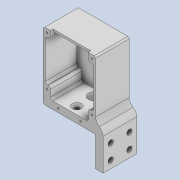
# Autodesk Inventor part: 0008-10-051 Cutie Priza
Saved by Autodesk Inventor 2020 (Build 240168000, 168)
## iProperties
Created: 2021-03-10
Part Number: 0008-10-051 Cutie Priza
Material: Generic
Document SubType Name: Modeling
Designer: Iulian Bors
Density: 1 g/cm^3
Appearance: Default
Description: Cutie priza
Mass: 164.87 g
Surface Area: 428.639 cm^2
Volume: 164.87 cm^3
Author: Iulian Bors
Subject: 051
Autodesk Inventor part; units mm, degrees
ref_plane "YZ Plane" through (0, 0, 0) normal (1, 0, 0) x (0, 1, 0)
ref_plane "XZ Plane" through (0, 0, 0) normal (0, 1, 0) x (-1, 0, 0)
ref_plane "XY Plane" through (0, 0, 0) normal (0, 0, 1) x (1, 0, 0)
sketch "Sketch1" plane through (0, 0, 0) normal (0, 0, 1) x (1, 0, 0)
  line L0 (-35, 45) -> (35, 45)
  line L1 (35, 45) -> (35, -45)
  line L2 (35, -45) -> (-35, -45)
  line L3 (-35, -45) -> (-35, 45)
  point P0 (0, 0)
  point P1 (0, 45)
  point P2 (-35, 0)
  dimension "d0" = 70
  dimension "d1" = 90
  constraints: 8 end point, 2 midpoint, 2 parallel, 1 horizontal, 1 horizontal alignment, 1 perpendicular, 1 vertical alignment
  measures "d0" distance of L0.start L0.end
  measures "d1" distance of L0.end L1.end
extrude "Extrusion1" add sketch "Sketch1" along normal blind 45
sketch "Sketch2" plane through (0, 0, 45) normal (0, 0, 1) x (1, 0, 0)
  line L0 (-25.3, 42) -> (25.3, 42)
  line L1 (25.3, 42) -> (25.3, -35)
  line L2 (25.3, -35) -> (-25.3, -35)
  line L3 (-25.3, -35) -> (-25.3, 42)
  line L4 (-35, 45) -> (-35, -45) projected
  line L5 (35, -45) -> (35, 45) projected
  line L6 (-35, -45) -> (35, -45) projected
  line L7 (35, 45) -> (-35, 45) projected
  point P0 (0, 0)
  dimension "d4" = 9.7
  dimension "d5" = 9.7
  dimension "d6" = 10
  dimension "d7" = 3
  constraints: 8 end point, 2 parallel, 1 horizontal, 1 perpendicular
  measures "d4" distance between parallel lines of L4 L3
  measures "d5" distance between parallel lines of L5 L1
  measures "d6" distance between parallel lines of L6 L2
  measures "d7" distance between parallel lines of L0 L7
extrude "Extrusion2" cut sketch "Sketch2" against normal blind 42 contours L0 L1 L2 L3
sketch "Sketch3" plane through (-35, 45, 0) normal (0, 1, 0) x (1, 0, 0)
  line L0 (60.3, -45) -> (9.7, -45)
  line L1 (9.7, -45) -> (9.7, -41.5)
  line L2 (9.7, -41.5) -> (60.3, -41.5)
  line L3 (60.3, -41.5) -> (60.3, -45)
  line L4 (9.7, -45) -> (9.7, -3) projected
  line L5 (60.3, -45) -> (60.3, -3) projected
  line L6 (70, -45) -> (0, -45) projected
  point P0 (35, 0)
  dimension "d10" = 3.5
  constraints: 8 end point, 3 collinear, 2 parallel, 1 horizontal, 1 perpendicular
  measures "d10" distance of L0.end L1.end
extrude "Extrusion3" cut sketch "Sketch3" against normal up to surface (3 mm away)
sketch "Sketch5" plane through (0, 0, 45) normal (0, 0, 1) x (1, 0, 0)
  line L0 (-33, 45) -> (-25, 45)
  line L1 (-25, 45) -> (25, 45)
  line L2 (25, 45) -> (33, 45)
  line L3 (33, 45) -> (35, 43)
  line L4 (35, 43) -> (35, -43)
  line L5 (35, -43) -> (33, -45)
  line L6 (33, -45) -> (-33, -45)
  line L7 (-33, -45) -> (-35, -43)
  line L8 (-35, -43) -> (-35, 43)
  line L9 (-35, 43) -> (-33, 45)
  line L10 (-25, -30) -> (-25, 45)
  line L11 (25, -30) -> (-25, -30)
  line L12 (25, 45) -> (25, -30)
  circle A0 centre (-30, 40) radius 2
  circle A1 centre (30, -25) radius 2
  circle A2 centre (-15, -40) radius 2
  circle A3 centre (15, -40) radius 2
  circle A4 centre (30, 40) radius 2
  circle A5 centre (-30, -25) radius 2
  line L13 (14.15, -21.6) -> (14.15, 28.85)
  arc A6 (14.15, 28.85) -> (11.65, 31.35) centre (11.65, 28.85) ccw
  line L14 (11.65, 31.35) -> (-12.5, 31.35)
  arc A7 (-12.5, 31.35) -> (-15, 28.85) centre (-12.5, 28.85) ccw
  line L15 (-15, 28.85) -> (-15, -21.6)
  arc A8 (-15, -21.6) -> (-12.5, -24.1) centre (-12.5, -21.6) ccw
  line L16 (-12.5, -24.1) -> (11.65, -24.1)
  arc A9 (11.65, -24.1) -> (14.15, -21.6) centre (11.65, -21.6) ccw
  circle A10 centre (20.135, 3.655) radius 2
  circle A11 centre (-19.865, 3.655) radius 2
  point P0 (0, 0)
  constraints: 34 end point, 12 centre point, 8 point on circle, 7 horizontal, 6 vertical, 48 other
hole "Hole2" at (-30, 40, 45) at (30, 40, 45) at (30, -25, 45) at (15, -40, 45) at (-15, -40, 45) at (-30, -25, 45) direction (0, 0, -1) diameter 2.459 depth 30 tip angle 118 thread size "M3x0.5" class "6H" standard "ISO Metric profile"
sketch "Sketch6" plane through (-25.3, -35, 45) normal (0, 1, 0) x (1, 0, 0)
  line L0 (50.6, 0) -> (0, 0) projected
  line L1 (0, 0) -> (0, 42) projected
  line L2 (50.6, 0) -> (50.6, 42) projected
  point P0 (25.3, 45)
  point P1 (10, 10)
  point P2 (25.3, 10)
  point P3 (25.3, 0)
  dimension "d30" = 10
  dimension "d31" = 10
  constraints: 1 horizontal alignment, 1 midpoint, 1 vertical alignment
  measures "d30" distance from line of L0 point (10, 10)
  measures "d31" distance from line of L1 point (10, 10)
hole "Hole3" at (0, -35, 35) direction (0, -1, 0) diameter 6 end through all countersink diameter 12 countersink angle 90
sketch "Sketch8" plane through (35, -45, 0) normal (1, 0, 0) x (0, 0, -1)
  line L0 (-45, 10) -> (0, 10)
  line L1 (0, 10) -> (0, -40)
  line L2 (0, -40) -> (-45, -40)
  line L3 (-45, -40) -> (-45, 10)
  line L4 (0, 0) -> (-45, 0) projected
  line L5 (-45, 0) -> (-45, 90) projected
  line L6 (0, 0) -> (0, 90) projected
  circle A0 centre (-35, -10) radius 3.5
  circle A1 centre (-10, -10) radius 3.5
  circle A2 centre (-35, -30) radius 3.5
  circle A3 centre (-10, -30) radius 3.5
  point P0 (0, 45)
  dimension "d42" = 10
  dimension "d43" = 40
  dimension "d44" = 7
  dimension "d45" = 7
  dimension "d46" = 10
  dimension "d47" = 10
  dimension "d48" = 10
  dimension "d59" = 10
  constraints: 8 end point, 4 centre point, 2 collinear, 2 equal radius, 2 horizontal alignment, 2 parallel, 2 vertical alignment, 1 horizontal, 1 perpendicular
  measures "d42" distance between parallel lines of L4 L0
  measures "d43" distance between parallel lines of L4 L2
  measures "d44" diameter of A0
  measures "d45" diameter of A1
  measures "d46" distance from line of A0.centre L3
  measures "d47" distance from line of L1 A1.centre
  measures "d48" distance from line of L4 A0.centre
  measures "d59" distance from line of L2 A2.centre
extrude "Extrusion4" add sketch "Sketch8" along normal blind 10
fillet "Fillet1" radius 10 2 edges at (35, -35, 22.5) (45, -35, 22.5)
chamfer "Chamfer2" distance 2 angle 45 3 edges at (35, 45, 22.5) (-35, 45, 22.5) (-35, -45, 22.5)
sketch "Sketch9" plane through (-25.3, -35, 45) normal (0, 1, 0) x (1, 0, 0)
  circle A0 centre (25.3, 33) radius 7.5
  line L0 (50.6, 42) -> (0, 42) projected
  point P0 (25.3, 45)
  point P1 (25.3, 42)
  dimension "d55" = 15
  dimension "d56" = 9
  constraints: 1 centre point, 1 midpoint, 1 vertical alignment
  measures "d55" diameter of A0
  measures "d56" distance from line of A0.centre L0
extrude "Extrusion5" cut sketch "Sketch9" against normal through all
sketch "Sketch10" plane through (0, 0, 45) normal (0, 0, 1) x (1, 0, 0)
  line L0 (-32, 35) -> (32, 35)
  line L1 (32, 35) -> (32, -20)
  line L2 (32, -20) -> (-32, -20)
  line L3 (-32, -20) -> (-32, 35)
  line L4 (-25.3, -35) -> (-25.3, 45) projected
  line L5 (-35, 43) -> (-35, -43) projected
  circle A0 centre (-30, 40) radius 1.2295 projected
  circle A1 centre (-30, -25) radius 1.2295 projected
  point P0 (0, 0)
  point P1 (0, 35)
  point P2 (-32, 7.5)
  dimension "d60" = 3
  dimension "d61" = 5
  dimension "d62" = 5
  constraints: 8 end point, 2 midpoint, 2 parallel, 1 horizontal, 1 perpendicular, 1 vertical alignment
  measures "d60" distance between parallel lines of L5 L3
  measures "d61" distance from line of A0.centre L0
  measures "d62" distance from line of A1.centre L2
extrude "Extrusion6" cut sketch "Sketch10" against normal up to surface (42 mm away) contours L0 L4 L2 L3 | L0 L1 L2 L4
fillet "Fillet2" radius 3 11 edges at (-25.3, -20, 24) (-32, -20, 24) (-32, 35, 24) (-25.3, 35, 24) (25.3, 42, 22.25) (25.3, 35, 24) (32, 35, 24) (32, -20, 24) (25.3, -20, 24) (25.3, -35, 24) (-25.3, -35, 24)
equation "\"d5\" = d4"
body "Solid1"
